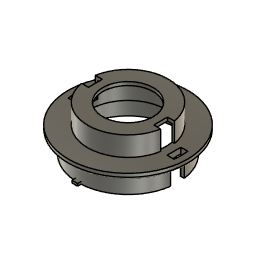
lamp_ring_shelves v4 (Autodesk Fusion 360 design; units mm, degrees)
Autodesk Fusion 360 part; units mm, degrees
note: some values were not read from the file. Set by a fixed rule: which sketch regions a step uses.
sketch "Sketch1" plane through (0, 0, 0) normal (0, 0, 1) x (1, 0, 0)
  circle A0 centre (0, 0) radius 43.5
  circle A1 centre (0, 0) radius 40.5
  dimension "d1" = 87
  dimension "d2" = 81
  constraint coincident A0.centre A1.centre
  constraint concentric A0 A1
  measures "d1" diameter of A0
  measures "d2" diameter of A1
extrude "Extrude1" add sketch "Sketch1" along normal blind 17 makes body 1
sketch "Sketch2" plane through (0, 0, 17) normal (0, 0, 1) x (-1, 0, 0)
  circle A0 centre (0, 0) radius 40.5
  circle A1 centre (0, 0) radius 43.5
  circle A2 centre (0, 0) radius 52
  circle A3 centre (0, 0) radius 33
  dimension "d5" = 104
  dimension "d6" = 66
  constraint coincident A0.centre A1.centre
  constraint concentric A2 A3
  measures "d5" diameter of A2
  measures "d6" diameter of A3
extrude "Extrude2" add sketch "Sketch2" along normal blind 5 contours A0 | A1 | A2 bodies 1
sketch "Sketch3" plane through (0, 0, 22) normal (0, 0, 1) x (-1, 0, 0)
  circle A0 centre (0, 0) radius 33
  circle A1 centre (0, 0) radius 52
  circle A2 centre (0, 0) radius 33
  circle A3 centre (0, 0) radius 35
  dimension "d9" = 70
  constraint coincident A0.centre A1.centre
  constraint concentric A2 A3
  measures "d9" diameter of A3
extrude "Extrude3" add sketch "Sketch3" along normal blind 14 contours A3 bodies 1
sketch "Sketch4" plane through (0, 0, 36) normal (0, 0, 1) x (-1, 0, 0)
  circle A0 centre (0, 0) radius 33
  circle A1 centre (0, 0) radius 35
  circle A2 centre (0, 0) radius 35
  circle A3 centre (0, 0) radius 22
  dimension "d12" = 44
  constraint concentric A0 A2
  constraint coincident A0.centre A1.centre
  measures "d12" diameter of A3
extrude "Extrude4" add sketch "Sketch4" along normal blind 3 contours A0 | A1 A2 bodies 1
sketch "Sketch5" plane through (0, 0, 39) normal (0, 0, 1) x (-1, 0, 0)
  circle A0 centre (0, 0) radius 22
  circle A1 centre (0, 0) radius 35
  line L0 (34.4819, 6) -> (34.4819, -6)
  line L1 (-34.4819, 6) -> (-28.4819, 6)
  line L2 (-28.4819, 6) -> (-28.4819, -6)
  line L3 (-28.4819, -6) -> (-34.4819, -6)
  line L4 (34.4819, 6) -> (28.4819, 6)
  line L5 (28.4819, 6) -> (28.4819, -6)
  line L6 (28.4819, -6) -> (34.4819, -6)
  line L7 (-34.4819, 6) -> (-28.4819, 6)
  line L8 (28.4819, 6) -> (34.4819, 6)
  line L9 (34.4819, -6) -> (28.4819, -6)
  line L10 (-28.4819, -6) -> (-34.4819, -6)
  arc A2 (-34.4819, 6) -> (-34.4819, -6) centre (0, 0) ccw
  arc A3 (34.4819, -6) -> (34.4819, 6) centre (0, 0) ccw
  dimension "d15" = 12
  dimension "d16" = 6
  dimension "d17" = 6
  constraint concentric A0 A2
  constraint horizontal L7
  constraint vertical L0
  constraint horizontal L9
  constraint coincident L0.end A2
  constraint horizontal L1
  constraint vertical L2
  constraint horizontal L3
  constraint coincident L2.end L9
  constraint horizontal L4
  constraint vertical L5
  constraint horizontal L6
  constraint collinear L7 L8
  constraint collinear L9 L10
  constraint concentric A2 A3
  measures "d15" distance of L7 L9
  measures "d16" distance of L1.start L1.end
  measures "d17" distance of L0.start L4.end
extrude "Extrude5" cut sketch "Sketch5" against normal blind 17 contours A1 L0 A3 | L0 L4 L5 L6 L8 L9 | A1 L1 L2 L3 L7 L10 A2 bodies 1
sketch "Sketch6" plane through (0, 0, 22) normal (0, 0, 1) x (-1, 0, 0)
  arc A0 (34.4819, 6) -> (-34.4819, 6) centre (0, 0) ccw
  line L0 (34.4819, 6) -> (32.45, 6)
  arc A1 (32.45, -6) -> (32.45, 6) centre (0, 0) ccw
  line L1 (32.45, -6) -> (34.4819, -6)
  arc A2 (-34.4819, -6) -> (34.4819, -6) centre (0, 0) ccw
  line L2 (-34.4819, -6) -> (-32.45, -6)
  arc A3 (-32.45, 6) -> (-32.45, -6) centre (0, 0) ccw
  line L3 (-32.45, 6) -> (-34.4819, 6)
  circle A4 centre (0, 0) radius 52
  line L4 (46.1113, -6) -> (40.1113, -6)
  line L5 (40.1113, -6) -> (40.1113, 6)
  line L6 (40.1113, 6) -> (46.1113, 6)
  line L7 (-46.1113, -6) -> (-40.1113, -6)
  line L8 (-40.1113, -6) -> (-40.1113, 6)
  line L9 (-40.1113, 6) -> (-46.1113, 6)
  line L10 (46.1113, -6) -> (40.1113, -6)
  line L11 (-46.1113, 6) -> (-40.1113, 6)
  line L12 (40.1113, 6) -> (46.1113, 6)
  line L13 (34.4819, -6) -> (32.45, -6)
  line L14 (-40.1113, -6) -> (-46.1113, -6)
  arc A5 (46.1113, -6) -> (46.1113, 6) centre (0, 0) ccw
  arc A6 (-46.1113, 6) -> (-46.1113, -6) centre (0, 0) ccw
  dimension "d20" = 93
  dimension "d21" = 12
  dimension "d22" = 6
  dimension "d23" = 6
  constraint coincident A0.centre A1.centre
  constraint horizontal L10
  constraint horizontal L11
  constraint coincident L9.end A5
  constraint horizontal L4
  constraint vertical L5
  constraint horizontal L6
  constraint coincident L5.end L11
  constraint horizontal L7
  constraint vertical L8
  constraint horizontal L9
  constraint collinear L10 L13
  constraint collinear L11 L12
  constraint concentric A5 A6
  measures "d20" diameter of A5
  measures "d21" distance of L10 L11
  measures "d22" distance of L4.start L4.end
  measures "d23" distance of L7.start L7.end
extrude "Extrude6" cut sketch "Sketch6" against normal blind 25 contours L4 L5 L6 L10 L12 A5 | L7 L8 L9 L11 L14 A6 bodies 1
sketch "Sketch7" plane through (0, 0, 0) normal (0, 0, -1) x (1, 0, 0)
  arc A0 (2.5, 46.4327) -> (-2.5, 46.4327) centre (0, 0) ccw
  arc A1 (-2.5, -46.4327) -> (2.5, -46.4327) centre (0, 0) ccw
  arc A2 (-2.5, -40.4228) -> (2.5, -40.4228) centre (0, 0) ccw
  arc A3 (2.5, 40.4228) -> (-2.5, 40.4228) centre (0, 0) ccw
  line L0 (2.5, 46.4327) -> (2.5, 40.4228)
  line L1 (2.5, -40.4228) -> (2.5, -46.4327)
  line L2 (-2.5, -46.4327) -> (-2.5, -40.4228)
  line L3 (-2.5, 40.4228) -> (-2.5, 46.4327)
  line L4 (43.0842, -6) -> (40.1113, -6)
  line L5 (40.1113, -6) -> (40.1113, -5.5978)
  arc A4 (-40.1113, -5.5978) -> (40.1113, -5.5978) centre (0, 0) ccw
  line L6 (-40.1113, -5.5978) -> (-40.1113, -6)
  line L7 (-40.1113, -6) -> (-43.0842, -6)
  arc A5 (-43.0842, -6) -> (43.0842, -6) centre (0, 0) ccw
  dimension "d26" = 93
  dimension "d27" = 5
  constraint coincident A0.centre A1.centre
  constraint vertical L2
  constraint vertical L0
  constraint coincident A1.start A0
  constraint concentric A0 A2
  constraint concentric A0 A1
  constraint coincident A2.end L0
  constraint concentric A2 A3
  constraint collinear L0 L1
  constraint collinear L2 L3
  measures "d26" diameter of A0
  measures "d27" distance of L0 L2
extrude "Extrude7" add sketch "Sketch7" against normal blind 2 separate body contours A0 A3 L0 L3 | A1 L1 L2 A5 | A2 L1 L2 A4 A5 makes body 2 at (-1.9446, -42.449, 0) makes body 3 at (1.9446, 42.449, 0)
fillet "Fillet1" radius 2 1 edges at (48.481, 18.804, 17) on bodies 1
sketch "Sketch8" plane through (0, 0, 17) normal (0, 0, -1) x (1, 0, 0)
  line L0 (43.0842, 6) -> (46.1113, 6)
  arc A0 (46.1113, -6) -> (46.1113, 6) centre (0, 0) ccw
  line L1 (46.1113, -6) -> (43.0842, -6)
  arc A1 (-43.0842, -6) -> (43.0842, -6) centre (0, 0) ccw
  line L2 (-43.0842, -6) -> (-46.1113, -6)
  arc A2 (-46.1113, 6) -> (-46.1113, -6) centre (0, 0) ccw
  line L3 (-46.1113, 6) -> (-43.0842, 6)
  arc A3 (43.0842, 6) -> (-43.0842, 6) centre (0, 0) ccw
  circle A4 centre (0, 0) radius 50
  circle A5 centre (0, 0) radius 46.5
  circle A6 centre (0, 0) radius 40.5
  dimension "d32" = 81
  constraint coincident A0.centre A1.centre
  measures "d32" diameter of A6
extrude "Extrude8" add sketch "Sketch8" along normal blind 2 contours L0 L3 A3 A5 | L1 A1 L2 A5 bodies 1
